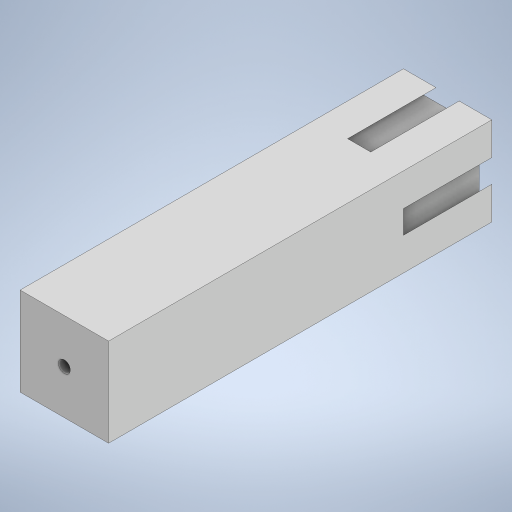
# Autodesk Inventor part: CarlaRescueRampeTeil1
Saved by Autodesk Inventor 2024 (Build 280153000, 153)
## iProperties
Created: 2024-01-16
Part Number: CarlaRescueRampeTeil1
Material: Generisch
Document SubType Name: Modeling
Designer: Robotik
Density: 1 g/cm^3
Appearance: Vorgabe
Author: Robotik
Autodesk Inventor part; units mm, degrees
ref_plane "YZ Plane" through (0, 0, 0) normal (1, 0, 0) x (0, 1, 0)
ref_plane "XZ Plane" through (0, 0, 0) normal (0, 1, 0) x (-1, 0, 0)
ref_plane "XY Plane" through (0, 0, 0) normal (0, 0, 1) x (1, 0, 0)
sketch "Skizze1" plane through (0, 0, 0) normal (0, 1, 0) x (-1, 0, 0)
  line L0 (25.085, 0) -> (-63.4246, 0)
  line L1 (0, 50.1146) -> (0, -66.9502)
  line L2 (15, 15) -> (-15, 15)
  line L3 (-15, 15) -> (-15, -15)
  line L4 (-15, -15) -> (15, -15)
  line L5 (15, -15) -> (15, 15)
  line L6 (15, 15) -> (-15, -15) construction
  line L7 (-15, 15) -> (15, -15) construction
  circle A0 centre (0, 0) radius 2
  dimension "d0" = 30
  dimension "d1" = 30
  dimension "d24" = 4
  constraints: 16 end point, 3 horizontal, 2 midpoint, 2 parallel, 2 vertical, 1 centre point, 1 coincident, 1 perpendicular
  measures "d0" distance of L4.end L2.start
  measures "d1" distance of L3.end L4.end
  measures "d24" diameter of A0
extrude "Extrusion1" add sketch "Skizze1" along normal blind 130
sketch "Skizze3" plane through (0, 130, 0) normal (0, 1, 0) x (1, 0, 0)
  line L0 (18.5438, 0) -> (-21.4353, 0) construction
  line L1 (-11, 7.5) -> (-11, -7.5)
  line L2 (-15, 15) -> (-15, -15) projected
  line L3 (15, 15) -> (-15, 15) projected
  line L4 (-11, 7.5) -> (-15, 3.5)
  line L5 (-11, -7.5) -> (-15, -3.5)
  line L6 (-15.2121, -3.7121) -> (-10.7, -8.2243)
  line L7 (-10.7, -8.2243) -> (-10.7, 8.2243)
  line L8 (-10.7, 8.2243) -> (-15.2121, 3.7121)
  line L9 (-15, -3.9243) -> (-15, 3.9243)
  line L10 (3.7121, -15.2121) -> (8.2243, -10.7)
  line L11 (8.2243, -10.7) -> (-8.2243, -10.7)
  line L12 (-8.2243, -10.7) -> (-3.7121, -15.2121)
  line L13 (3.9243, -15) -> (-3.9243, -15)
  line L14 (15.2121, 3.7121) -> (10.7, 8.2243)
  line L15 (10.7, 8.2243) -> (10.7, -8.2243)
  line L16 (10.7, -8.2243) -> (15.2121, -3.7121)
  line L17 (15, 3.9243) -> (15, -3.9243)
  line L18 (-3.7121, 15.2121) -> (-8.2243, 10.7)
  line L19 (-8.2243, 10.7) -> (8.2243, 10.7)
  line L20 (8.2243, 10.7) -> (3.7121, 15.2121)
  line L21 (-3.9243, 15) -> (3.9243, 15)
  point P0 (0, 0)
  point P1 (3.9243, 15)
  point P2 (-3.9243, 15)
  dimension "d11" = 4
  dimension "d12" = 15
  dimension "d13" = 7.5
  dimension "d14" = 45
  dimension "d15" = 45
  dimension "d18" = 0.3
  dimension "d22" = 360
  constraints: 40 end point, 12 point on line, 2 horizontal, 1 vertical, 43 other
  measures "d11" distance between parallel lines of L2 L1
  measures "d12" distance of L1.start L1.end
  measures "d13" distance from line of L3 L1.start
  measures "d14" angle of L2 L4
  measures "d15" angle of L2 L5
  measures "d18" distance between parallel lines of L5 L6
extrude "Extrusion3" cut sketch "Skizze3" against normal blind 30
fillet "Rundung1" radius 0.2 2 edges at (-15, 115, 3.9243) (-15, 115, -3.9243)
extrude "Extrusion4" cut sketch "Skizze1" along normal blind 6.7 contours A0 L1 L0 | L0 L1 A0 | L1 A0 L0 | L0 A0 L1
